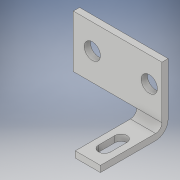
# Autodesk Inventor part: dsub37bracket_redraw
Saved by Autodesk Inventor 2017 (Build 210142000, 142)
## iProperties
Created: 2019-01-25
Part Number: dsub37bracket_redraw
Material: Generic
Document SubType Name: Modeling
Designer: Zara
Density: 1 g/cm^3
Appearance: Default
Sheet Metal Width: 0.000 in
Sheet Metal Length: 0.000 in
Sheet Metal Area: 0.000 in^2
Sheet Metal Rule: Default
Author: Zara
Autodesk Inventor part; units mm, degrees
ref_plane "YZ Plane" through (0, 0, 0) normal (1, 0, 0) x (0, 1, 0)
ref_plane "XZ Plane" through (0, 0, 0) normal (0, 1, 0) x (-1, 0, 0)
ref_plane "XY Plane" through (0, 0, 0) normal (0, 0, 1) x (1, 0, 0)
sketch "Sketch1" plane through (0, 0, 0) normal (0, 0, 1) x (1, 0, 0)
  line L0 (0, 0) -> (15.24, 0)
  line L1 (21.2852, 0) -> (21.2852, 12.5984)
  line L2 (21.2852, 12.5984) -> (0, 12.5984)
  line L3 (0, 12.5984) -> (0, 0)
  line L4 (15.24, 0) -> (15.24, -15.621)
  line L5 (15.24, -15.621) -> (21.2852, -15.621)
  line L6 (21.2852, -15.621) -> (21.2852, 0)
  line L7 (0, 0) -> (15.24, 0)
  dimension "d0" = 21.2852
  dimension "d1" = 12.5984
  dimension "d2" = 6.0452
  dimension "d3" = 15.621
  constraints: 16 end point, 3 parallel, 2 horizontal, 1 perpendicular
  measures "d0" distance of L1.end L2.end
  measures "d1" distance of L1.start L1.end
  measures "d2" distance of L4.end L5.end
  measures "d3" distance of L0.end L4.end
extrude "Extrusion1" add sketch "Sketch1" along normal blind 1.4986
sketch "Sketch2" plane through (0, 0, 1.4986) normal (0, 0, 1) x (1, 0, 0)
  circle A0 centre (4.572, 6.5532) radius 1.9558
  line L0 (21.2852, 12.5984) -> (0, 12.5984) projected
  line L1 (0, 12.5984) -> (0, 0) projected
  circle A1 centre (18.2626, 6.5532) radius 1.9558
  dimension "d6" = 3.9116
  dimension "d7" = 6.0452
  dimension "d8" = 4.572
  dimension "d11" = 13.6906
  constraints: 2 centre point, 1 horizontal, 2 other
  measures "d6" diameter of A0
  measures "d7" distance from line of A0.centre L0
  measures "d8" distance from line of L1 A0.centre
  measures "d11" distance of A0.centre A1.centre
extrude "Extrusion2" cut sketch "Sketch2" against normal blind 25.4
sketch "Sketch3" plane through (0, 0, 1.4986) normal (0, 0, 1) x (1, 0, 0)
  circle A0 centre (18.2626, -11.6332) radius 1.4478
  line L0 (15.24, -15.621) -> (21.2852, -15.621) projected
  line L1 (15.24, 0) -> (15.24, -15.621) projected
  circle A1 centre (18.2626, -7.6708) radius 1.4478
  line L2 (16.8148, -7.6708) -> (18.2626, -7.6708)
  line L3 (19.7104, -11.6332) -> (17.1196, -11.6332)
  point P0 (0, 0)
  dimension "d18" = 2.8956
  dimension "d19" = 3.9878
  dimension "d20" = 3.0226
  dimension "d26" = 3.9624
  constraints: 4 end point, 2 horizontal alignment, 2 vertical, 1 horizontal, 1 parallel, 5 other
  measures "d19" distance from line of point (18.263, -11.633) L0
  measures "d20" distance from line of point (18.263, -11.633) L1
  measures "d26" distance of L2.end point (18.263, -11.633)
extrude "Extrusion4" cut sketch "Sketch3" against normal blind 25.4
sketch "Sketch6" plane through (0, 0, 1.4986) normal (0, 0, 1) x (1, 0, 0)
  circle A0 centre (18.2626, -7.6708) radius 1.4478 projected
  circle A1 centre (18.2626, -11.6332) radius 1.4478 projected
  line L0 (16.8148, -7.6708) -> (19.7104, -7.6708)
  line L1 (19.7104, -7.6708) -> (19.7104, -11.6332)
  line L2 (19.7104, -11.6332) -> (16.8148, -11.6332)
  line L3 (16.8148, -11.6332) -> (16.8148, -7.6708)
  point P0 (0, 0)
  constraints: 8 end point, 2 horizontal alignment, 2 parallel, 1 horizontal, 1 perpendicular, 2 other
extrude "Extrusion5" cut sketch "Sketch6" against normal blind 25.4 contours L1 A1 L3 A0 | A0 L0 | L2 A1 picked at (18.2044, -8.1499) picked at (18.4337, -11.182)
sketch "Sketch16" plane through (0, 0, 1.4986) normal (0, 0, 1) x (1, 0, 0)
  line L0 (0, 0) -> (15.24, 0) projected
  line L1 (15.24, 0) -> (21.2852, 0)
  line L2 (21.2852, -15.621) -> (21.2852, 12.5984) projected
  constraints: 2 end point, 1 horizontal, 1 point on line
bend part "Bend Part2" radius 1.4986 angle 90 line through (15.24, 0, 1.4986) along (1, 0, 0) centre toward (0, 0, 1) moving side (0, -1, 0) both sides no
equation "\"BendRadius\" = Thickness"
equation "\"BendReliefWidth\" = Thickness"
equation "\"BendReliefDepth\" = 0.5 * Thickness"
equation "\"CornerReliefSize\" = 4 * Thickness"
equation "\"MinimumRemnant\" = 2 * Thickness"
equation "\"TransitionRadius\" = BendRadius"
equation "\"JacobiRadiusSize\" = Thickness"
equation "\"GapSize\" = Thickness"
equation "\"Thickness\" = 3.048"
body "Solid1"
